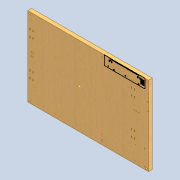
# Autodesk Inventor part: 0005-10-001-Batiu
Saved by Autodesk Inventor 2020 (Build 240168000, 168)
## iProperties
Created: 2020-12-18
Part Number: 0005-10-001-Batiu
Material: Generic
Document SubType Name: Modeling
Designer: Iulian Bors
Density: 1 g/cm^3
Appearance: Yellow Pine - Solid Stained Light Low Gloss
Mass: 5352.4 g
Surface Area: 5922.17 cm^2
Volume: 5352.4 cm^3
Author: Iulian Bors
Subject: 001
Autodesk Inventor part; units mm, degrees
ref_plane "YZ Plane" through (0, 0, 0) normal (1, 0, 0) x (0, 1, 0)
ref_plane "XZ Plane" through (0, 0, 0) normal (0, 1, 0) x (-1, 0, 0)
ref_plane "XY Plane" through (0, 0, 0) normal (0, 0, 1) x (1, 0, 0)
sketch "Sketch1" plane through (0, 0, 0) normal (0, 0, 1) x (1, 0, 0)
  line L0 (-365, 210) -> (365, 210)
  line L1 (365, 210) -> (365, -210)
  line L2 (365, -210) -> (-365, -210)
  line L3 (-365, -210) -> (-365, 210)
  point P0 (0, 0)
  point P1 (-365, 0)
  point P2 (0, 210)
  dimension "d0" = 730
  dimension "d1" = 420
  constraints: 8 end point, 2 midpoint, 2 parallel, 1 horizontal, 1 horizontal alignment, 1 perpendicular, 1 vertical alignment
  measures "d0" distance of L0.start L0.end
  measures "d1" distance of L2.end L0.start
extrude "Extrusion1" add sketch "Sketch1" along normal blind 20
sketch "Sketch2" plane through (0, 0, 20) normal (0, 0, 1) x (1, 0, 0)
  line L0 (-365, 210) -> (-365, -210) projected
  line L1 (-255, 30) -> (-245, 30) construction
  line L2 (-255, 27.75) -> (-245, 27.75)
  line L3 (-245, 32.25) -> (-255, 32.25)
  arc A0 (-255, 32.25) -> (-255, 27.75) centre (-255, 30) ccw
  arc A1 (-245, 27.75) -> (-245, 32.25) centre (-245, 30) ccw
  line L4 (365, 210) -> (-365, 210) projected
  line L5 (-255, 10) -> (-245, 10) construction
  line L6 (-255, 7.75) -> (-245, 7.75)
  line L7 (-245, 12.25) -> (-255, 12.25)
  arc A2 (-255, 12.25) -> (-255, 7.75) centre (-255, 10) ccw
  arc A3 (-245, 7.75) -> (-245, 12.25) centre (-245, 10) ccw
  point P0 (0, 0)
  point P1 (-250, 30)
  point P2 (-250, 10)
  dimension "d5" = 4.5
  dimension "d6" = 10
  dimension "d7" = 115
  dimension "d9" = 180
  dimension "d12" = 20
  constraints: 16 end point, 8 point on circle, 4 centre point, 4 tangent, 1 horizontal, 1 midpoint, 1 parallel, 1 vertical, 12 other
  measures "d5" distance between parallel lines of L2 L3
  measures "d6" distance of L1.start L1.end
  measures "d7" distance from line of point (-250, 30) L0
  measures "d9" distance from line of L4 point (-250, 30)
  measures "d12" distance of L2.start L6.start
extrude "Extrusion2" cut sketch "Sketch2" against normal through all
sketch "Sketch3" plane through (0, 0, 20) normal (0, 0, 1) x (1, 0, 0)
  circle A0 centre (-261.807, 82) radius 2.25
  circle A1 centre (-261.807, 117) radius 2.25
  circle A2 centre (-277.807, 82) radius 2.25
  circle A3 centre (-277.807, 117) radius 2.25
  line L0 (-284.807, 122) -> (-254.807, 122)
  line L1 (-254.807, 122) -> (-254.807, 77)
  line L2 (-254.807, 77) -> (-284.807, 77)
  line L3 (-284.807, 77) -> (-284.807, 122)
  circle A4 centre (-261.807, -108) radius 2.25
  circle A5 centre (-261.807, -73) radius 2.25
  circle A6 centre (-277.807, -108) radius 2.25
  circle A7 centre (-277.807, -73) radius 2.25
  line L4 (-284.807, -68) -> (-254.807, -68)
  line L5 (-254.807, -68) -> (-254.807, -113)
  line L6 (-254.807, -113) -> (-284.807, -113)
  line L7 (-284.807, -113) -> (-284.807, -68)
  circle A8 centre (276.227, 82) radius 2.25
  circle A9 centre (276.227, 117) radius 2.25
  circle A10 centre (260.227, 82) radius 2.25
  circle A11 centre (260.227, 117) radius 2.25
  line L8 (253.227, 122) -> (283.227, 122)
  line L9 (283.227, 122) -> (283.227, 77)
  line L10 (283.227, 77) -> (253.227, 77)
  line L11 (253.227, 77) -> (253.227, 122)
  line L12 (291.227, -60) -> (275.227, -60) construction
  line L13 (275.227, -60) -> (275.227, -95) construction
  line L14 (275.227, -95) -> (291.227, -95) construction
  line L15 (291.227, -95) -> (291.227, -60) construction
  line L16 (291.227, -57.5) -> (291.227, -62.5) construction
  line L17 (288.977, -57.5) -> (288.977, -62.5)
  line L18 (293.477, -62.5) -> (293.477, -57.5)
  arc A12 (293.477, -57.5) -> (288.977, -57.5) centre (291.227, -57.5) ccw
  arc A13 (288.977, -62.5) -> (293.477, -62.5) centre (291.227, -62.5) ccw
  line L19 (291.227, -92.5) -> (291.227, -97.5) construction
  line L20 (288.977, -92.5) -> (288.977, -97.5)
  line L21 (293.477, -97.5) -> (293.477, -92.5)
  arc A14 (293.477, -92.5) -> (288.977, -92.5) centre (291.227, -92.5) ccw
  arc A15 (288.977, -97.5) -> (293.477, -97.5) centre (291.227, -97.5) ccw
  line L22 (275.227, -92.5) -> (275.227, -97.5) construction
  line L23 (272.977, -92.5) -> (272.977, -97.5)
  line L24 (277.477, -97.5) -> (277.477, -92.5)
  arc A16 (277.477, -92.5) -> (272.977, -92.5) centre (275.227, -92.5) ccw
  arc A17 (272.977, -97.5) -> (277.477, -97.5) centre (275.227, -97.5) ccw
  line L25 (275.227, -57.5) -> (275.227, -62.5) construction
  line L26 (272.977, -57.5) -> (272.977, -62.5)
  line L27 (277.477, -62.5) -> (277.477, -57.5)
  arc A18 (277.477, -57.5) -> (272.977, -57.5) centre (275.227, -57.5) ccw
  arc A19 (272.977, -62.5) -> (277.477, -62.5) centre (275.227, -62.5) ccw
  line L28 (365, -210) -> (365, 210) projected
  line L29 (-365, -210) -> (365, -210) projected
  circle A20 centre (291.227, -95) radius 2.25
  circle A21 centre (291.227, -60) radius 2.25
  circle A22 centre (275.227, -60) radius 2.25
  circle A23 centre (275.227, -95) radius 2.25
  point P0 (0, 0)
  point P1 (272.977, -60)
  point P2 (277.477, -60)
  point P3 (277.477, -95)
  point P4 (272.977, -95)
  point P5 (288.977, -95)
  point P6 (293.477, -95)
  point P7 (293.477, -60)
  point P8 (288.977, -60)
  dimension "d23" = 35
  dimension "d24" = 16
  dimension "d25" = 5
  dimension "d26" = 4.5
  dimension "d29" = 115
  dimension "d30" = 73.773
  constraints: 64 end point, 24 centre point, 18 tangent, 16 point on circle, 7 horizontal, 7 parallel, 6 vertical, 5 coincident, 5 equal radius, 4 midpoint, 3 equal length, 2 perpendicular, 2 point on line, 36 other
  measures "d23" distance of L14.end L12.start
  measures "d24" distance of L13.end L14.end
  measures "d25" distance of L16.start L16.end
  measures "d26" distance between parallel lines of L17 L18
  measures "d29" distance between parallel lines of L29 L14
  measures "d30" distance between parallel lines of L15 L28
extrude "Extrusion3" cut sketch "Sketch3" against normal through all contours A12 L18 A21 L17 | A21 L18 A13 L17 | A21 | A14 L21 A20 L20 | A20 L21 A15 L20 | A20 | A16 L24 A23 L23 | A23 L24 A17 L23 | A23 | A18 L27 A22 L26 | A22 L27 A19 L26 | A22
move faces "Move2" translate (90, 0, 0) faces at (-365, 70, 13.3333)
pattern_linear "Rectangular Pattern1" count 2 spacing 190 along (0, 1, 0) count 2 spacing 538.034 along (-1, 0, 0) of "Extrusion3"
sketch "Sketch4" plane through (0, 0, 20) normal (0, 0, 1) x (1, 0, 0)
  line L0 (-265, 200) -> (355, 200) construction
  line L1 (355, 200) -> (355, -200) construction
  line L2 (355, -200) -> (-265, -200) construction
  line L3 (-265, -200) -> (-265, 200) construction
  arc A0 (-255, 12.25) -> (-255, 7.75) centre (-255, 10) ccw construction
  line L4 (-255, 12.25) -> (-245, 12.25) construction
  arc A1 (-245, 7.75) -> (-245, 12.25) centre (-245, 10) ccw construction
  line L5 (-245, 7.75) -> (-255, 7.75) construction
  line L6 (-245, 27.75) -> (-255, 27.75) construction
  arc A2 (-255, 32.25) -> (-255, 27.75) centre (-255, 30) ccw construction
  line L7 (-255, 32.25) -> (-245, 32.25) construction
  arc A3 (-245, 27.75) -> (-245, 32.25) centre (-245, 30) ccw construction
  line L8 (-275, 210) -> (-275, -210) construction
  line L9 (-275, -210) -> (365, -210) construction
  line L10 (365, -210) -> (365, 210) construction
  line L11 (365, 210) -> (-275, 210) construction
  point P0 (0, 0)
  point P1 (45, 200)
  point P2 (45, 210)
  point P3 (-265, 0)
  point P4 (-365, 0)
  dimension "d56" = 10
  dimension "d57" = 10
  dimension "d58" = 10
  dimension "d59" = 10
  constraints: 8 end point, 4 coincident, 2 midpoint, 2 parallel, 1 horizontal, 1 horizontal alignment, 1 perpendicular, 1 vertical alignment
  measures "d56" distance between parallel lines of L8 L3
  measures "d57" distance between parallel lines of L0 L11
  measures "d58" distance between parallel lines of L10 L1
  measures "d59" distance between parallel lines of L9 L2
hole "Hole1" at (-265, 200, 20) at (355, 200, 20) at (355, -200, 20) at (-265, -200, 20) direction (0, 0, -1) diameter 8 end through all
sketch "Sketch5" plane through (0, 0, 20) normal (0, 0, 1) x (1, 0, 0)
  line L0 (357, 70.5491) -> (365, 70.5491)
  line L1 (365, 70.5491) -> (365, 58.8141)
  line L2 (365, 58.8141) -> (357, 58.8141)
  line L3 (357, 58.8141) -> (357, 70.5491)
  line L4 (365, 101.5791) -> (357, 101.5791)
  line L5 (357, 101.5791) -> (357, 113.3141)
  line L6 (357, 113.3141) -> (365, 113.3141)
  line L7 (365, 113.3141) -> (365, 101.5791)
  point P0 (0, 0)
  point P1 (361, 64.6816)
  point P2 (361, 107.4466)
  point P3 (361, 70.5491)
  point P4 (361, 113.3141)
  point P5 (357, 64.6816)
  point P6 (357, 107.4466)
  constraints: 16 end point, 4 horizontal, 4 midpoint, 4 vertical, 2 horizontal alignment, 2 vertical alignment, 8 other
hole "Hole2" at (361, 64.6816, 20) at (361, 107.4466, 20) direction (0, 0, -1) diameter 4 end through all
sketch "Sketch6" plane through (0, 0, 20) normal (0, 0, 1) x (1, 0, 0)
  line L0 (110, -140) -> (130, -140)
  line L1 (130, -140) -> (130, -210)
  line L2 (130, -210) -> (110, -210)
  line L3 (110, -210) -> (110, -140)
  line L4 (130, 175) -> (110, 175)
  line L5 (110, 175) -> (110, 210)
  line L6 (110, 210) -> (130, 210)
  line L7 (130, 210) -> (130, 175)
  point P0 (0, 0)
  point P1 (120, 192.5)
  point P2 (120, -190)
  point P3 (120, -160)
  point P4 (120, 175)
  point P5 (130, 192.5)
  point P6 (120, -210)
  dimension "d67" = 20
  dimension "d68" = 20
  constraints: 16 end point, 4 horizontal, 4 vertical, 3 midpoint, 3 vertical alignment, 1 horizontal alignment, 8 other
  measures "d67" distance of point (120, -210) point (120, -190)
  measures "d68" distance from line of L0 point (120, -160)
hole "Hole3" at (120, 192.5, 20) at (120, -190, 20) at (120, -160, 20) direction (0, 0, -1) diameter 8 end through all
sketch "Sketch7" plane through (0, 0, 20) normal (0, 0, 1) x (1, 0, 0)
  line L0 (276.09, 31.1) -> (326.09, 31.1) projected
  line L1 (284.7184, 41.4) -> (317.4616, 41.4) projected
  line L2 (-275, -210) -> (365, -210) projected
  line L3 (365, -210) -> (365, 210) projected
  point P0 (0, 0)
  point P1 (288.5, 35)
  point P2 (301, 35)
  point P3 (313.5, 35)
  dimension "d76" = 241.1
  dimension "d77" = 245
  dimension "d78" = 38.91
  dimension "d79" = 50
  dimension "d80" = 12.5
  dimension "d81" = 12.5
  dimension "d82" = 51.5
  constraints: 2 horizontal alignment
  measures "d76" distance between parallel lines of L2 L0
  measures "d77" distance from line of L2 point (301, 35)
  measures "d78" distance from line of L3 L0.end
  measures "d79" distance of L0.start L0.end
  measures "d80" distance of point (313.5, 35) point (301, 35)
  measures "d81" distance of point (301, 35) point (288.5, 35)
  measures "d82" distance from line of L3 point (313.5, 35)
hole "Hole4" at (288.5, 35, 20) at (301, 35, 20) at (313.5, 35, 20) direction (0, 0, -1) diameter 4.5 end through all
sketch "Sketch8" plane through (0, 0, 20) normal (0, 0, 1) x (1, 0, 0)
  circle A0 centre (342.5, -198) radius 1.6078
  circle A1 centre (294.3339, -122.0389) radius 1.6
  circle A2 centre (294.004, -196.7238) radius 1.6078
  circle A3 centre (342.5, -115.0463) radius 1.6078
  point P0 (0, 0)
  constraints: 4 centre point, 8 other
hole "Hole5" at (342.5, -198, 20) at (294.004, -196.7238, 20) at (294.3339, -122.0389, 20) at (342.5, -115.0463, 20) direction (0, 0, -1) diameter 2.459 end through all thread size "M3x0.5" class "6H" standard "ISO Metric profile"
sketch "Sketch9" plane through (0, 0, 20) normal (0, 0, 1) x (1, 0, 0)
  circle A0 centre (152, 169.4) radius 1.5
  circle A1 centre (243, 169.4) radius 1.5
  circle A2 centre (181, 165.9) radius 3
  circle A3 centre (312, 165.9) radius 3
  circle A4 centre (163, 199) radius 1.7
  circle A5 centre (313, 199) radius 1.7
  line L0 (311.5, 210) -> (345, 210)
  line L1 (345, 210) -> (345, 160.9)
  line L2 (345, 160.9) -> (130, 160.9)
  line L3 (130, 160.9) -> (130, 210)
  line L4 (130, 210) -> (161.5, 210)
  line L5 (161.5, 210) -> (161.5, 206.5)
  arc A6 (161.5, 206.5) -> (164.5, 206.5) centre (163, 206.5) ccw
  line L6 (164.5, 206.5) -> (164.5, 210)
  line L7 (164.5, 210) -> (168.5, 210)
  line L8 (168.5, 210) -> (168.5, 206.5)
  arc A7 (168.5, 206.5) -> (171.5, 206.5) centre (170, 206.5) ccw
  line L9 (171.5, 206.5) -> (171.5, 210)
  line L10 (171.5, 210) -> (175.5, 210)
  line L11 (175.5, 210) -> (175.5, 206.5)
  arc A8 (175.5, 206.5) -> (178.5, 206.5) centre (177, 206.5) ccw
  line L12 (178.5, 206.5) -> (178.5, 210)
  line L13 (178.5, 210) -> (182.5, 210)
  line L14 (182.5, 210) -> (182.5, 206.5)
  arc A9 (182.5, 206.5) -> (185.5, 206.5) centre (184, 206.5) ccw
  line L15 (185.5, 206.5) -> (185.5, 210)
  line L16 (185.5, 210) -> (189.5, 210)
  line L17 (189.5, 210) -> (189.5, 206.5)
  arc A10 (189.5, 206.5) -> (192.5, 206.5) centre (191, 206.5) ccw
  line L18 (192.5, 206.5) -> (192.5, 210)
  line L19 (192.5, 210) -> (196.5, 210)
  line L20 (196.5, 210) -> (196.5, 206.5)
  arc A11 (196.5, 206.5) -> (199.5, 206.5) centre (198, 206.5) ccw
  line L21 (199.5, 206.5) -> (199.5, 210)
  line L22 (199.5, 210) -> (203.5, 210)
  line L23 (203.5, 210) -> (203.5, 206.5)
  arc A12 (203.5, 206.5) -> (206.5, 206.5) centre (205, 206.5) ccw
  line L24 (206.5, 206.5) -> (206.5, 210)
  line L25 (206.5, 210) -> (210.5, 210)
  line L26 (210.5, 210) -> (210.5, 206.5)
  arc A13 (210.5, 206.5) -> (213.5, 206.5) centre (212, 206.5) ccw
  line L27 (213.5, 206.5) -> (213.5, 210)
  line L28 (213.5, 210) -> (217.5, 210)
  line L29 (217.5, 210) -> (217.5, 206.5)
  arc A14 (217.5, 206.5) -> (220.5, 206.5) centre (219, 206.5) ccw
  line L30 (220.5, 206.5) -> (220.5, 210)
  line L31 (220.5, 210) -> (224.5, 210)
  line L32 (224.5, 210) -> (224.5, 206.5)
  arc A15 (224.5, 206.5) -> (227.5, 206.5) centre (226, 206.5) ccw
  line L33 (227.5, 206.5) -> (227.5, 210)
  line L34 (227.5, 210) -> (231.5, 210)
  line L35 (231.5, 210) -> (231.5, 206.5)
  arc A16 (231.5, 206.5) -> (234.5, 206.5) centre (233, 206.5) ccw
  line L36 (234.5, 206.5) -> (234.5, 210)
  line L37 (234.5, 210) -> (238.5, 210)
  line L38 (238.5, 210) -> (238.5, 206.5)
  arc A17 (238.5, 206.5) -> (241.5, 206.5) centre (240, 206.5) ccw
  line L39 (241.5, 206.5) -> (241.5, 210)
  line L40 (241.5, 210) -> (245.5, 210)
  line L41 (245.5, 210) -> (245.5, 206.5)
  arc A18 (245.5, 206.5) -> (248.5, 206.5) centre (247, 206.5) ccw
  line L42 (248.5, 206.5) -> (248.5, 210)
  line L43 (248.5, 210) -> (252.5, 210)
  line L44 (252.5, 210) -> (252.5, 206.5)
  arc A19 (252.5, 206.5) -> (255.5, 206.5) centre (254, 206.5) ccw
  line L45 (255.5, 206.5) -> (255.5, 210)
  line L46 (255.5, 210) -> (259.5, 210)
  line L47 (259.5, 210) -> (259.5, 206.5)
  arc A20 (259.5, 206.5) -> (262.5, 206.5) centre (261, 206.5) ccw
  line L48 (262.5, 206.5) -> (262.5, 210)
  line L49 (262.5, 210) -> (266.5, 210)
  line L50 (266.5, 210) -> (266.5, 206.5)
  arc A21 (266.5, 206.5) -> (269.5, 206.5) centre (268, 206.5) ccw
  line L51 (269.5, 206.5) -> (269.5, 210)
  line L52 (269.5, 210) -> (273.5, 210)
  line L53 (273.5, 210) -> (273.5, 206.5)
  arc A22 (273.5, 206.5) -> (276.5, 206.5) centre (275, 206.5) ccw
  line L54 (276.5, 206.5) -> (276.5, 210)
  line L55 (276.5, 210) -> (280.5, 210)
  line L56 (280.5, 210) -> (280.5, 206.5)
  arc A23 (280.5, 206.5) -> (283.5, 206.5) centre (282, 206.5) ccw
  line L57 (283.5, 206.5) -> (283.5, 210)
  line L58 (283.5, 210) -> (287.5, 210)
  line L59 (287.5, 210) -> (287.5, 206.5)
  arc A24 (287.5, 206.5) -> (290.5, 206.5) centre (289, 206.5) ccw
  line L60 (290.5, 206.5) -> (290.5, 210)
  line L61 (290.5, 210) -> (294.5, 210)
  line L62 (294.5, 210) -> (294.5, 206.5)
  arc A25 (294.5, 206.5) -> (297.5, 206.5) centre (296, 206.5) ccw
  line L63 (297.5, 206.5) -> (297.5, 210)
  line L64 (297.5, 210) -> (301.5, 210)
  line L65 (301.5, 210) -> (301.5, 206.5)
  arc A26 (301.5, 206.5) -> (304.5, 206.5) centre (303, 206.5) ccw
  line L66 (304.5, 206.5) -> (304.5, 210)
  line L67 (304.5, 210) -> (308.5, 210)
  line L68 (308.5, 210) -> (308.5, 206.5)
  arc A27 (308.5, 206.5) -> (311.5, 206.5) centre (310, 206.5) ccw
  line L69 (311.5, 206.5) -> (311.5, 210)
  arc A28 (337.5, 173.95) -> (340.5, 173.95) centre (339, 173.95) ccw
  line L70 (340.5, 173.95) -> (340.5, 196.95)
  arc A29 (340.5, 196.95) -> (337.5, 196.95) centre (339, 196.95) ccw
  line L71 (337.5, 196.95) -> (337.5, 173.95)
  arc A30 (330.5, 173.95) -> (333.5, 173.95) centre (332, 173.95) ccw
  line L72 (333.5, 173.95) -> (333.5, 196.95)
  arc A31 (333.5, 196.95) -> (330.5, 196.95) centre (332, 196.95) ccw
  line L73 (330.5, 196.95) -> (330.5, 173.95)
  line L74 (326.5, 173.95) -> (326.5, 196.95)
  arc A32 (326.5, 196.95) -> (323.5, 196.95) centre (325, 196.95) ccw
  line L75 (323.5, 196.95) -> (323.5, 173.95)
  arc A33 (323.5, 173.95) -> (326.5, 173.95) centre (325, 173.95) ccw
  line L76 (320.5, 199) -> (318, 199)
  line L77 (318, 199) -> (318, 192)
  line L78 (318, 192) -> (320.5, 192)
  line L79 (320.5, 192) -> (320.5, 199)
  line L80 (308, 192) -> (308, 199)
  line L81 (308, 199) -> (305.5, 199)
  line L82 (305.5, 199) -> (305.5, 192)
  line L83 (305.5, 192) -> (308, 192)
  line L84 (170.5, 199) -> (168, 199)
  line L85 (168, 199) -> (168, 192)
  line L86 (168, 192) -> (170.5, 192)
  line L87 (170.5, 192) -> (170.5, 199)
  line L88 (158, 192) -> (158, 199)
  line L89 (158, 199) -> (155.5, 199)
  line L90 (155.5, 199) -> (155.5, 192)
  line L91 (155.5, 192) -> (158, 192)
  point P0 (0, 0)
  constraints: 184 end point, 60 vertical, 56 point on circle, 34 centre point, 32 horizontal, 188 other
hole "Hole6" at (243, 169.4, 20) at (152, 169.4, 20) direction (0, 0, -1) diameter 4 end through all
equation "\"d81\" = d80"
body "Solid1"
